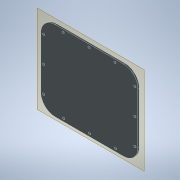
# Autodesk Inventor part: Крышка фонаря 1
Saved by Autodesk Inventor 2021 (Build 250183000, 183)
## iProperties
Created: 2020-12-11
Part Number: Крышка фонаря 1
Material: Чугун, серый
Document SubType Name: Modeling
Designer: Тимоха
Mass: 3305.12 g
Surface Area: 1921.8 cm^2
Volume: 462.254 cm^3
Density: 7.15 g/cm^3
Appearance: Чугун серый
Author: Тимоха
Autodesk Inventor part; units mm, degrees
ref_plane "YZ Plane" through (0, 0, 0) normal (1, 0, 0) x (0, 1, 0)
ref_plane "XZ Plane" through (0, 0, 0) normal (0, 1, 0) x (-1, 0, 0)
ref_plane "XY Plane" through (0, 0, 0) normal (0, 0, 1) x (1, 0, 0)
ref_plane "РабПлоскость1" through (0, 0, 0) normal (0, 0, 1) x (1, 0, 0)
sketch "Эскиз1" plane through (0, 0, 0) normal (0, 0, 1) x (1, 0, 0)
  circle A0 centre (-91.8879, 130) radius 4 projected
  circle A1 centre (-0.944, 130) radius 4 projected
  circle A2 centre (90, 130) radius 4 projected
  circle A3 centre (159.9555, 91.8872) radius 4 projected
  circle A4 centre (160, 0.944) radius 4 projected
  circle A5 centre (160, -90) radius 4 projected
  circle A6 centre (91.8879, -130) radius 4 projected
  circle A7 centre (0.944, -130) radius 4 projected
  circle A8 centre (-90, -130) radius 4 projected
  circle A9 centre (-159.9555, -91.8872) radius 4 projected
  circle A10 centre (-160, -0.944) radius 4 projected
  circle A11 centre (-160, 90) radius 4 projected
  arc A12 (-170, -90) -> (-120, -140) centre (-120, -90) ccw projected
  line L0 (-120, -140) -> (120, -140) projected
  arc A13 (120, -140) -> (170, -90) centre (120, -90) ccw projected
  line L1 (170, -90) -> (170, 90) projected
  arc A14 (170, 90) -> (120, 140) centre (120, 90) ccw projected
  line L2 (120, 140) -> (-120, 140) projected
  arc A15 (-120, 140) -> (-170, 90) centre (-120, 90) ccw projected
  line L3 (-170, 90) -> (-170, -90) projected
  line L4 (120, -120) -> (-120, -120) projected
  arc A16 (-150, -90) -> (-120, -120) centre (-120, -90) ccw projected
  line L5 (-150, -90) -> (-150, 90) projected
  arc A17 (-120, 120) -> (-150, 90) centre (-120, 90) ccw projected
  line L6 (-120, 120) -> (120, 120) projected
  arc A18 (150, 90) -> (120, 120) centre (120, 90) ccw projected
  line L7 (150, 90) -> (150, -90) projected
  arc A19 (120, -120) -> (150, -90) centre (120, -90) ccw projected
  point P0 (0, 0)
extrude "Выдавливание1" add sketch "Эскиз1" along normal blind 5 contours L3 A15 L2 A14 L1 A13 L0 A12 | L4 A16 L5 A17 L6 A18 L7 A19
